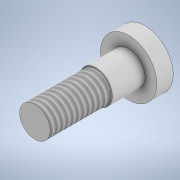
# Autodesk Inventor part: M2_6-2_8-5_3
Saved by Autodesk Inventor 2020.4 (Build 244396000, 396)
## iProperties
Created: 2021-09-23
Part Number: M2_6-2_8-5_3
Material: 一般
Document SubType Name: Modeling
Designer: Masato
Density: 1 g/cm^3
Appearance: 既定
Author: Masato
Autodesk Inventor part; units mm, degrees
ref_plane "YZ Plane" through (0, 0, 0) normal (1, 0, 0) x (0, 1, 0)
ref_plane "XZ Plane" through (0, 0, 0) normal (0, 1, 0) x (-1, 0, 0)
ref_plane "XY Plane" through (0, 0, 0) normal (0, 0, 1) x (1, 0, 0)
sketch "スケッチ1" plane through (0, 0, 0) normal (0, 1, 0) x (-1, 0, 0)
  line L0 (0, 0) -> (2.4, 0)
  line L1 (2.4, 0) -> (2.4, 1.4)
  line L2 (2.4, 1.4) -> (1.4, 1.4)
  line L3 (1.4, 1.4) -> (1.4, 4.2)
  line L4 (1.4, 4.2) -> (1.3, 4.2)
  line L5 (1.3, 4.2) -> (1.3, 9.4)
  line L6 (1.3, 9.4) -> (0, 9.4)
  line L7 (0, 9.4) -> (0, 0)
  dimension "d0" = 1.3
  dimension "d1" = 5.2
  dimension "d2" = 2.8
  dimension "d3" = 1.4
  dimension "d4" = 2.4
  dimension "d5" = 1.4
  constraints: 16 end point, 7 perpendicular, 1 horizontal
  measures "d0" distance of L5.end L6.end
  measures "d1" distance of L4.end L5.end
  measures "d2" distance of L2.end L3.end
  measures "d3" distance of L0.end L1.end
  measures "d4" distance of L0.start L0.end
  measures "d5" horizontal distance of L0.start L2.end
revolve "回転1" add sketch "スケッチ1" angle 360 about axis through (0, 0, 9.4) along (0, 0, -1)
thread "ねじ1" size "M2.6x0.45" class "6g" standard "ANSI Metric M Profile" full length
